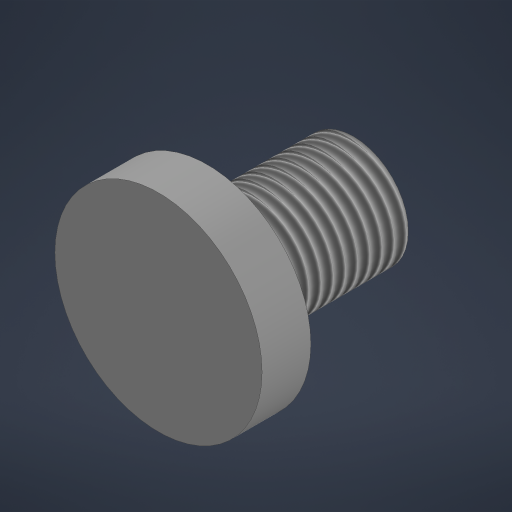
# Autodesk Inventor part: vida
Saved by Autodesk Inventor 2023 (Build 270158030, 158C)
## iProperties
Created: 2023-03-11
Part Number: vida
Material: Generic
Document SubType Name: Modeling
Designer: Monster
Density: 1 g/cm^3
Appearance: Default
Author: Monster
Autodesk Inventor part; units mm, degrees
ref_plane "YZ Plane" through (0, 0, 0) normal (1, 0, 0) x (0, 1, 0)
ref_plane "XZ Plane" through (0, 0, 0) normal (0, 1, 0) x (-1, 0, 0)
ref_plane "XY Plane" through (0, 0, 0) normal (0, 0, 1) x (1, 0, 0)
sketch "Sketch1" plane through (0, 0, 0) normal (0, 0, 1) x (1, 0, 0)
  circle A0 centre (0, 0) radius 4.25
  dimension "d0" = 8.5
  constraints: 1 centre point, 1 coincident
  measures "d0" diameter of A0
extrude "Extrusion1" add sketch "Sketch1" along normal blind 2
sketch "Sketch2" plane through (0, 0, 0) normal (0, 0, -1) x (-1, 0, 0)
  circle A0 centre (0, 0) radius 2.25
  dimension "d3" = 4.5
  constraints: 1 centre point, 1 coincident
  measures "d3" diameter of A0
extrude "Extrusion2" add sketch "Sketch2" along normal blind 6
sketch "Sketch3" plane through (0, 0, 2) normal (0, 0, 1) x (1, 0, 0)
  circle A0 centre (0, 0) radius 2.25 projected
  circle A1 centre (0, 0) radius 4.25 projected
  line L0 (-4.25, 0) -> (-2.125, 3.6806)
  line L1 (-2.125, 3.6806) -> (2.125, 3.6806)
  line L2 (2.125, 3.6806) -> (4.25, 0)
  line L3 (4.25, 0) -> (2.125, -3.6806)
  line L4 (2.125, -3.6806) -> (-2.125, -3.6806)
  line L5 (-2.125, -3.6806) -> (-4.25, 0)
  constraints: 12 end point, 1 coincident, 15 other
extrude "Extrusion3" add sketch "Sketch3" against normal blind 2 contours L2 A1 | A1 L3 | L1 A1 | A1 L4 | L0 A1 | A1 L5
thread "Thread2" size "M3x0.5" class "6g" standard "ANSI Metric M Profile" length 6
body "Solid1"
